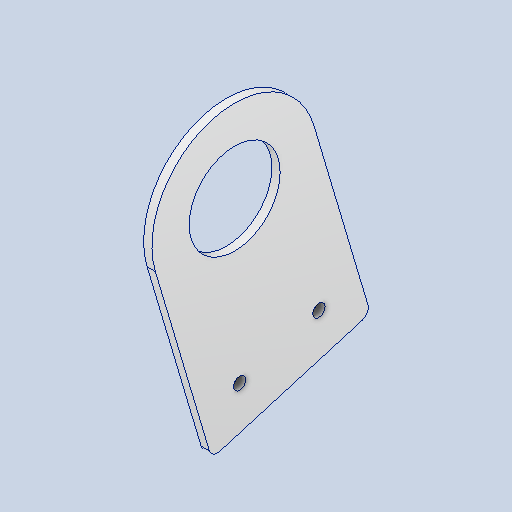
# Autodesk Inventor part: dribl-v1-Plate-13
Saved by Autodesk Inventor 2025.2 (Build 292293000, 293)
## iProperties
Created: 2025-01-16
Part Number: dribl-v1-Plate-13
Material: アルミニウム 6061
Document SubType Name: Modeling
Designer: haruy
Density: 2.7 g/cm^3
Appearance: アルミニウム - フラット
Author: haruy
Autodesk Inventor part; units mm, degrees
ref_plane "YZ Plane" through (0, 0, 0) normal (1, 0, 0) x (0, 1, 0)
ref_plane "XZ Plane" through (0, 0, 0) normal (0, 1, 0) x (-1, 0, 0)
ref_plane "XY Plane" through (0, 0, 0) normal (0, 0, 1) x (1, 0, 0)
sketch "スケッチ1" plane through (0, 0, 0) normal (1, 0, 0) x (0, 1, 0)
  circle A0 centre (75.1066, 546.1804) radius 20
  line L0 (398.3077, -642.9996) -> (12.4603, 659.0318)
  line L1 (-81.8954, -654.6507) -> (-61.8954, -654.6507)
  line L2 (-6.7154, 653.3493) -> (379.132, -648.6822)
  line L3 (23.4023, 551.7179) -> (69.424, 565.3561)
  line L4 (34.7675, 513.3665) -> (80.7892, 527.0047)
  circle A1 centre (75.1066, 546.1804) radius 11
  line L5 (12.4603, 659.0318) -> (-6.7154, 653.3493)
  circle A2 centre (35.8315, 544.9714) radius 1.5
  circle A3 centre (41.514, 525.7956) radius 1.5
  point P0 (0, 0)
  point P1 (-384.8954, -222.3173)
  dimension "d0" = 40
  dimension "d1" = 28
  dimension "d2" = 22
  dimension "d3" = 106
  dimension "d4" = 3
  dimension "d5" = 3
  dimension "d6" = 10
  dimension "d7" = 10
  dimension "d8" = 10
  dimension "d9" = 20
  constraints: 12 end point, 4 centre point, 2 perpendicular, 2 point on circle, 2 point on line, 2 tangent, 1 coincident
  measures "d0" diameter of A0
  measures "d1" distance from line of L0 A0.centre
  measures "d2" diameter of A1
  measures "d3" distance between parallel lines of L3 L5
  measures "d4" diameter of A2
  measures "d5" diameter of A3
  measures "d6" distance from line of A2.centre L3
  measures "d7" distance from line of A2.centre L2
  measures "d8" distance from line of A3.centre L2
  measures "d9" distance of A3.centre A2.centre
extrude "押し出し1" add sketch "スケッチ1" against normal blind 2 contours A0 | A0 L4 L0 L3 | L0 L4 L2 L3
fillet "フィレット1" radius 2 2 edges at (-1, 23.4023, 551.7179) (-1, 34.7675, 513.3665)
equation "\"d7\" = d6"
equation "\"d8\" = d6"
